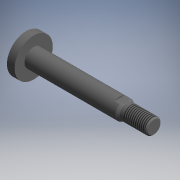
# Autodesk Inventor part: CDQSB25-40DM(1_0)_ROD
Saved by Autodesk Inventor 2017.3 (Build 213256000, 256)
## iProperties
Part Number: CDQSB25-40DM(1_0)_ROD
Material: Generic
Catalog Web Link: www.cadenas.de
Description: CQS/CDQS ROD-Compact Cylinder:Standard Type Double Acting,Single Rod
Vendor: SMC
Document SubType Name: Modeling
Designer: partserver
Manufacturer: SMC
Mass: 10.6809 g
Surface Area: 41.9113 cm^2
Volume: 10.6809 cm^3
Density: 1 g/cm^3
Appearance: PSOLRGB-128-128-128
Category: PARTsolutions
Company: SMC
Title: CDQSB25-40DM_ROD
Author: Cadenas PARTsolutions
Comments: Compact Cylinder:Standard Type Double Acting,Single Rod
PSOL_IDENT_0: {$CADENAS_DATA\23d-libs\smc_jp\actuator\compact_cylinder\cqs\cqs\parts\cqs_rod.prj},241 {VTYP=3D},{N
PSOL_IDENT_1: B=CDQSB25-40DM(1_0)_ROD},{LINA=CDQSB25-40DM_ROD},{NN=CQS/CDQS ROD},{DATE=29.10.2021 06:14:24},{GEOMD
PSOL_IDENT_2: ATE=13.07.2018 01:24:00},{VERSION=},{LINEID=40},{WBVAR=TYPE,MOUNT,MAGNET,STROKE,STOP,BODY,AUTOSWITCH
PSOL_IDENT_3: ,THREAD},{WBNUMERIC=STROKE}  {NB=CDQSB25-40DM(1_0)_ROD},{LINA=CDQSB25-40DM_ROD},{KT=DUMMY},{TYPE=},{
PSOL_IDENT_4: TP=A},{BORE=25},{MOUNT=B},{MAGNET=D},{STROKE=40},{STROKEX2=40},{STOP=1},{ACTION=(D) Double acting},{
PSOL_IDENT_5: BODY=M},{BODYX='','(-) Standard (Rod end female thread)','C','(C) With rubber bumper','M','(M) Rod e
PSOL_IDENT_6: nd male thread','F','(F) Boss on head side','CM','(CM) With rubber bumper & Rod end male thread','FC'
PSOL_IDENT_7: ,'(FC) Boss on head side & With rubber bumper','FM','(FM) Boss on head side & Rod end male thread','
PSOL_IDENT_8: FCM','(FCM) Boss on head side & With rubber bumper & Rod end male thread'},{ORDER=CDQSB25-40DM},{AUT
PSOL_IDENT_9: OSWITCH=},{AUTOSWITCHX='','(-) Without autoswitch','-M9NV','M9NV','-M9PV','M9PV','-M9BV','M9BV','-M9
PSOL_IDENT_10: N','M9N','-M9P','M9P','-M9B','M9B','-M9NWV','M9NWV','-M9PWV','M9PWV','-M9BWV','M9BWV','-M9NW','M9NW'
PSOL_IDENT_11: ,'-M9PW','M9PW','-M9BW','M9BW','-M9NAV','M9NAV','-M9PAV','M9PAV','-M9BAV','M9BAV','-M9NA','M9NA','-M
PSOL_IDENT_12: 9PA','M9PA','-M9BA','M9BA','-A96V','A96V','-A93V','A93V','-A90V','A90V','-A96','A96','-A93','A93','-
PSOL_IDENT_13: A90','A90','-P3DWA','P3DWA','-P3DWASC','P3DWASC','-P3DWASE','P3DWASE'},{THREAD=0},{B=32.5},{BB1=22.5
PSOL_IDENT_14: },{BB2=32.5},{BB3=44.0},{L=5.0},{LL1=5.0},{LL2=15.0},{C=12},{D=12},{H=M6x1.0},{HRA=6},{HRP=1.0},{K=1
PSOL_IDENT_15: 0},{KA=5.0},{C1=15},{L1=22.5},{L11=22.5},{L12=32.5},{MM=M10x1.25},{MMRA=10},{MMRP=1.25},{X=17.5}
NB: CDQSB25-40DM(1_0)_ROD
NN: CQS/CDQS ROD
NT: Compact Cylinder:Standard Type Double Acting,Single Rod
NBSYN: $ORDER.($STOP._$THREAD.)_ROD
LINA: CDQSB25-40DM_ROD
CATALOG: SMC (JP
TYPE: (-) None
BORE: 25
MOUNT: (B) Through-hole/Both ends tapped common (Standard)
MAGNET: (D) With magnet
STROKE: 40
STOP: Manufacturable stroke
ACTION: (D) Double acting
BODY: (M) Rod end male thread
AUTOSWITCH: (-) Without autoswitch
THREAD: on
B: 32.5
L: 5
C: 12
D: 12
H: M6x1.0
K: 10
KA: 5
C1: 15
L1: 22.5
MM: M10x1.25
MMRA: 10
MMRP: 1.25
X: 17.5
SUPPLIER: SMC
ARTICLENO: CDQSB25-40DM(1_0)_ROD
BOMINFO: CDQSB25-40DM_ROD
CREATOR: CADENAS GmbH
Autodesk Inventor part; units mm, degrees
sketch "Sketch_3" plane through (0, 0, 0) normal (0, 0, 1) x (1, 0, 0)
  line L0 (61.25, 0) -> (-22.5, 0)
  line L1 (-22.5, 0) -> (-22.5, 4.233)
  line L2 (-22.5, 4.233) -> (-21.733, 5)
  line L3 (-21.733, 5) -> (-5, 5)
  line L4 (-5, 5) -> (-3.2679, 6)
  line L5 (-3.2679, 6) -> (56.25, 6)
  line L6 (56.25, 6) -> (56.25, 12.5)
  line L7 (56.25, 12.5) -> (61.25, 12.5)
  line L8 (61.25, 12.5) -> (61.25, 0)
  line L9 (61.25, 0) -> (-22.5, 0)
  constraints: 20 end point
revolve "Revolution1" add sketch "Sketch_3" angle 360 about axis through (61.25, 0, 0) along (1, 0, 0)
thread "Thread1" size "M10x1.25" class "6g" standard "ISO Metric profile" length 14.233
sketch "Sketch_7" plane through (0, 0, 0) normal (1, 0, 0) x (0, 0, -1)
  circle A0 centre (0, 0) radius 12
  line L0 (-5, 7) -> (-5, -7)
  line L1 (-5, -7) -> (5, -7)
  line L2 (5, -7) -> (5, 7)
  line L3 (5, 7) -> (-5, 7)
  constraints: 8 end point, 1 centre point
extrude "Extrusion1" cut sketch "Sketch_7" against normal blind 5
ref_plane "ROD_BODY_XY" through (0, 0, 0) normal (1, 0, 0) x (0, 0, -1)
ref_plane "ROD_BODY_YZ" through (0, 0, 0) normal (0, 0, -1) x (0, 1, 0)
ref_plane "ROD_BODY_ZX" through (0, 0, 0) normal (0, 1, 0) x (1, 0, 0)
ref_plane "ROD_NUT_XY" through (-22.5, 0, 0) normal (-1, 0, 0) x (0, 0, -1)
ref_plane "ROD_NUT_YZ" through (-22.5, 0, 0) normal (0, 0, -1) x (0, -1, 0)
ref_plane "ROD_NUT_ZX" through (-22.5, 0, 0) normal (0, -1, 0) x (-1, 0, 0)
body "Solid1"
